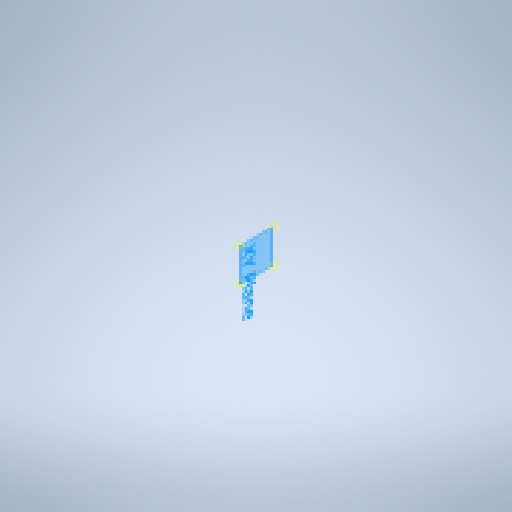
# Autodesk Inventor part: longerScrew
Saved by Autodesk Inventor 2023 (Build 270158000, 158)
## iProperties
Created: 2023-03-19
Part Number: longerScrew
Material: Generic
Document SubType Name: Modeling
Designer: shrey
Density: 1 g/cm^3
Appearance: Default
Author: shrey
Autodesk Inventor part; units mm, degrees
ref_plane "YZ Plane" through (0, 0, 0) normal (1, 0, 0) x (0, 1, 0)
ref_plane "XZ Plane" through (0, 0, 0) normal (0, 1, 0) x (-1, 0, 0)
ref_plane "XY Plane" through (0, 0, 0) normal (0, 0, 1) x (1, 0, 0)
ref_plane "Work Plane1" through (-22, 18, -9.9035) normal (0, -1, 0) x (0, 0, -1)
sketch "Sketch1" plane through (-22, 18, -9.9035) normal (0, -1, 0) x (0, 0, -1)
  spline S0 degree 3 poles (41.079, 4.2882) (41.1539, 4.1612) (41.2485, 4.0469) (41.4813, 3.8418) (41.6216, 3.7561) (41.9369, 3.6326) (42.1108, 3.5998) (42.4706, 3.6003) (42.653, 3.6369) (42.99, 3.7773) (43.142, 3.8786) (43.3765, 4.1113) (43.4651, 4.2329) (43.6017, 4.5018) (43.648, 4.6478) (43.6753, 4.8356) (43.6793, 4.8732) (43.683, 4.9311) (43.6838, 4.9515) (43.6846, 4.9887) (43.6846, 5.0055) (43.684, 5.0419) (43.6833, 5.0615) (43.6802, 5.1152) (43.6769, 5.1493) (43.6596, 5.2804) (43.6366, 5.3761) (43.5593, 5.5938) (43.4972, 5.7121) (43.331, 5.9422) (43.2234, 6.0494) (42.9677, 6.2329) (42.819, 6.3043) (42.4931, 6.3953) (42.3177, 6.4104) (41.96, 6.3744) (41.7817, 6.3196) (41.4606, 6.1462) (41.3201, 6.0307) (41.1088, 5.775) (41.0318, 5.6432) (40.9361, 5.3938) (40.9083, 5.2815) (40.8908, 5.1364) (40.8882, 5.1057) (40.8856, 5.0572) (40.8849, 5.0395) (40.8844, 5.0069) (40.8844, 4.9919) (40.885, 4.9591) (40.8856, 4.9412) (40.8884, 4.891) (40.8913, 4.8587) (40.9067, 4.735) (40.9271, 4.645) (40.9875, 4.4636) (41.0287, 4.3733) (41.079, 4.2882) knots 0 0 0 0 0.044326 0.044326 0.093383 0.093383 0.146079 0.146079 0.201356 0.201356 0.255644 0.255644 0.300529 0.300529 0.346168 0.346168 0.357482 0.357482 0.363591 0.363591 0.368644 0.368644 0.374518 0.374518 0.384776 0.384776 0.41421 0.41421 0.454101 0.454101 0.499414 0.499414 0.548537 0.548537 0.600928 0.600928 0.656444 0.656444 0.710644 0.710644 0.75624 0.75624 0.790854 0.790854 0.800101 0.800101 0.805408 0.805408 0.809903 0.809903 0.81526 0.81526 0.824988 0.824988 0.852648 0.852648 0.88238 0.88238 0.88238 0.88238 projected
  point P0 (-9.9035, 22)
  point P1 (41.079, 4.2882)
extrude "Extrusion1" add sketch "Sketch1" against normal blind 24.6
sketch "Sketch2" plane through (-17, 42.6, -52.188) normal (0, 1, 0) x (1, 0, 0)
  circle A0 centre (0, 0) radius 2.95
  point P0 (17, -52.188)
  dimension "d2" = 5.9
  constraints: 1 centre point
  measures "d2" diameter of A0
extrude "Extrusion2" add sketch "Sketch2" along normal blind 2.4
chamfer "Chamfer1" distance 2 angle 30 1 edges at (-19.95, 45, -52.188) measured on face at (-16.264, 45, -53.3107)
body "Solid1"
